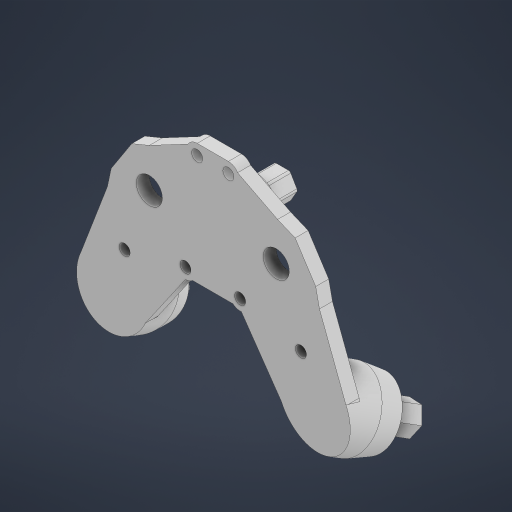
# Autodesk Inventor part: Neck_Baseplate_V2
Saved by Autodesk Inventor 2024 (Build 280153000, 153)
## iProperties
Created: 2025-09-27
Part Number: Neck_Baseplate_V2
Material: Generic
Document SubType Name: Modeling
Designer: kevin
Density: 1 g/cm^3
Appearance: Default
Author: kevin
Autodesk Inventor part; units mm, degrees
sketch "Sketch1" plane through (0, 0, 0) normal (0, 0, 1) x (1, 0, 0)
  line L0 (-6.0622, -7.1524) -> (-3.0311, -1.9024) projected
  line L1 (-3.0311, -1.9024) -> (3.0311, -1.9024) projected
  line L2 (3.0311, -1.9024) -> (6.0622, -7.1524) projected
  line L3 (6.0622, -7.1524) -> (3.0311, -12.4024) projected
  line L4 (3.0311, -12.4024) -> (-3.0311, -12.4024) projected
  line L5 (-3.0311, -12.4024) -> (-6.0622, -7.1524) projected
  circle A0 centre (0, -7.1524) radius 8.6602 projected
  line L6 (2.9156, -2.1024) -> (5.8312, -7.1524)
  line L7 (5.8312, -7.1524) -> (2.9156, -12.2024)
  line L8 (2.9156, -12.2024) -> (-2.9156, -12.2024)
  line L9 (-2.9156, -12.2024) -> (-5.8312, -7.1524)
  line L10 (-5.8312, -7.1524) -> (-2.9156, -2.1024)
  line L11 (-2.9156, -2.1024) -> (2.9156, -2.1024)
  point P0 (0, 0)
  dimension "d0" = 10.1
  constraints: 12 end point, 1 coincident, 1 parallel, 13 other
  measures "d0" distance between parallel lines of L8 L11
ref_plane "Work Plane1" through (-12.6537, -14.3928, -10.5) normal (0, 0, -1) x (0, 1, 0)
extrude "Extrusion1" add sketch "Sketch1" against normal up to surface (10.5 mm away) contours L6 L7 L8 L9 L10 L11
sketch "Sketch3" plane through (0, 0, 0) normal (0, 0, 1) x (1, 0, 0)
  circle A0 centre (0, -7.1524) radius 11.4859 projected
  arc A1 (11.152, -14.925) -> (11.152, 0.6202) centre (0, -7.1524) ccw projected
  circle A2 centre (0, -7.1524) radius 13.5934
  point P0 (0, 0)
  point P1 (11.152, 0.6202)
  point P2 (11.152, -14.925)
  constraints: 1 centre point, 1 coincident
extrude "Extrusion3" add sketch "Sketch3" along normal blind 11 contours A0 | A2 A1
ref_plane "Work Plane2" through (-43.2893, -53.3143, -8.1555) normal (0.2018432, 0.4641283, 0.862464) x (0.9791415, -0.1165411, -0.1664337)
sketch "Sketch5" plane through (-43.2893, -53.3143, -8.1555) normal (0.2018432, 0.4641283, 0.862464) x (0.9791415, -0.1165411, -0.1664337)
  line L0 (-6.0622, -7.1524) -> (-3.0311, -1.9024) projected
  line L1 (-3.0311, -1.9024) -> (3.0311, -1.9024) projected
  line L2 (3.0311, -1.9024) -> (6.0622, -7.1524) projected
  line L3 (6.0622, -7.1524) -> (3.0311, -12.4024) projected
  line L4 (3.0311, -12.4024) -> (-3.0311, -12.4024) projected
  line L5 (-3.0311, -12.4024) -> (-6.0622, -7.1524) projected
  circle A0 centre (0, -7.1524) radius 8.6602 projected
  line L6 (-2.9156, -12.2024) -> (-5.8312, -7.1524)
  line L7 (-5.8312, -7.1524) -> (-2.9156, -2.1024)
  line L8 (-2.9156, -2.1024) -> (2.9156, -2.1024)
  line L9 (2.9156, -2.1024) -> (5.8312, -7.1524)
  line L10 (5.8312, -7.1524) -> (2.9156, -12.2024)
  line L11 (2.9156, -12.2024) -> (-2.9156, -12.2024)
  point P0 (34.8157, 43.9226)
  dimension "d13" = 10.1
  constraints: 12 end point, 1 coincident, 1 parallel, 13 other
  measures "d13" distance between parallel lines of L8 L11
ref_plane "Work Plane3" through (-55.9189, -67.2082, -9.8974) normal (-0.2018432, -0.4641283, -0.862464) x (0.0232659, 0.8780678, -0.4779703)
extrude "Extrusion4" add sketch "Sketch5" against normal up to surface (10.5 mm away) contours L6 L7 L8 L9 L10 L11
fillet "Fillet1" radius 1 12 edges at (-47.2527, -57.2572, -11.1933) (-50.225, -61.3517, -8.2943) (-47.4877, -66.1257, -6.3658) (-41.5431, -57.9368, -12.1638) (-38.8058, -62.7108, -10.2354) (-41.7781, -66.8053, -7.3363) (-2.9156, -2.1024, -5.25) (-5.8312, -7.1524, -5.25) (-2.9156, -12.2024, -5.25) (2.9156, -2.1024, -5.25) (5.8312, -7.1524, -5.25) (2.9156, -12.2024, -5.25)
sketch "Sketch6" plane through (-43.2893, -53.3143, -8.1555) normal (0.2018432, 0.4641283, 0.862464) x (0.9791415, -0.1165411, -0.1664337)
  circle A0 centre (0, -7.1524) radius 11.4859 projected
  arc A1 (-11.152, 0.6202) -> (-11.152, -14.925) centre (0, -7.1524) ccw projected
  circle A2 centre (0, -7.1524) radius 13.5934
  point P0 (34.8157, 43.9226)
  point P1 (-11.152, -14.925)
  point P2 (-11.152, 0.6202)
  constraints: 1 centre point, 1 coincident
extrude "Extrusion5" add sketch "Sketch6" along normal blind 25.4 contours A0 | A2 A1
chamfer "Chamfer3" distance 2 angle 80 1 edges at (-32.7172, -67.7191, -2.8779) measured on face at (-43.6596, -66.527, -0.9586)
chamfer "Chamfer4" distance 2.75 angle 45 1 edges at (-34.2972, -66.5238, -3.1514)
chamfer "Chamfer5" distance 5 angle 45 1 edges at (-11.152, 0.6202, 0)
mirror "Mirror1" about plane through (0, 0, 0) normal (1, 0, 0) of "Extrusion4", "Extrusion5", "Chamfer4", "Chamfer3"
sketch "Sketch7" plane through (0, -7.1524, 11) normal (0, 0, 1) x (1, 0, 0)
  line L0 (62, -125.9339) -> (62, 49.4211) projected
  line L1 (-62, -125.9339) -> (62, -125.9339) projected
  line L2 (-62, 49.4211) -> (-62, -125.9339) projected
  line L3 (62, 49.4211) -> (-62, 49.4211) projected
  circle A0 centre (-35.0416, -115.806) radius 4 projected
  circle A1 centre (-0.3458, -115.806) radius 4 projected
  circle A2 centre (34.35, -115.806) radius 4 projected
  circle A3 centre (0, -77.5722) radius 2.1 projected
  circle A4 centre (-11, -67.3741) radius 2.1 projected
  circle A5 centre (11, -67.3741) radius 2.1 projected
  circle A6 centre (-6.25, 18.8827) radius 2.1 projected
  circle A7 centre (33.6286, -26.3451) radius 2.1 projected
  circle A8 centre (5.75, 18.8827) radius 2.1 projected
  circle A9 centre (-34.1286, -26.3451) radius 2.1 projected
  circle A10 centre (24.1373, -1.8845) radius 6.75 projected
  circle A11 centre (-24.6373, -1.8845) radius 6.75 projected
  circle A12 centre (-10.7484, -20.4549) radius 2.1 projected
  circle A13 centre (10.2484, -20.4549) radius 2.1 projected
  ellipse E0 centre (-38.3289, -40.6533) end of major axis (-25.8633, -46.0745) minor radius 11.7238 projected
  line L4 (0, -181.6265) -> (0, 141.5467)
  circle A14 centre (-6.25, 18.8827) radius 4.1
  circle A15 centre (5.75, 18.8827) radius 4.1
  line L5 (-6.25, 22.9827) -> (5.75, 22.9827)
  circle A16 centre (-24.6373, -1.8845) radius 8.75 construction
  line L6 (-9.7714, 20.9827) -> (-24.6373, 13.1086)
  line L7 (-24.6373, 13.1086) -> (-31.3873, 10.3122)
  line L8 (-31.3873, 10.3122) -> (-39.29, -1.8845)
  line L9 (-39.29, -1.8845) -> (-40.7219, -8.6345)
  line L10 (-40.7219, -8.6345) -> (-50.9767, -35.6799)
  arc A17 (-10.7484, -24.5549) -> (-8.0196, -23.5149) centre (-10.7484, -20.4549) ccw
  arc A18 (7.5196, -23.5149) -> (10.7288, -24.5267) centre (10.2484, -20.4549) ccw
  line L11 (24.6373, 13.1086) -> (31.3873, 10.3122)
  line L12 (31.3873, 10.3122) -> (39.29, -1.8845)
  line L13 (39.29, -1.8845) -> (40.7219, -8.6345)
  line L14 (40.7219, -8.6345) -> (50.9767, -35.6799)
  ellipse E1 centre (38.3289, -40.6533) end of major axis (25.8633, -46.0745) minor radius 11.7238 projected
  line L15 (-26.3694, -47.081) -> (-10.7484, -24.5549)
  line L16 (-8.0196, -23.5149) -> (7.5196, -23.5149)
  line L17 (26.3694, -47.081) -> (10.7288, -24.5267)
  line L18 (-9.7714, 20.9827) -> (18.0265, 20.9827) construction
  line L19 (9.2714, 20.9827) -> (24.6373, 13.1086)
  circle A19 centre (-24.6373, -1.8845) radius 5
  circle A20 centre (24.1373, -1.8845) radius 5
  point P0 (0, 7.1524)
  point P1 (10.7484, -24.5549)
  point P2 (26.3694, -47.081)
  dimension "d28" = 2
  dimension "d29" = 2
  dimension "d30" = 2
  dimension "d31" = 2
  dimension "d32" = 2
  dimension "d37" = 10
  dimension "d38" = 10
  constraints: 32 end point, 8 point on circle, 7 centre point, 7 symmetric about line, 2 coincident, 2 horizontal, 2 point on line, 1 tangent, 1 vertical, 7 other
  measures "d28" radial gap between concentric circles of A6 A14
  measures "d29" radial gap between concentric circles of A8 A15
  measures "d30" radial gap between concentric circles of A11 A16
  measures "d31" radial gap between concentric circles of A12 A17
  measures "d32" radial gap between concentric circles of A13 A18
  measures "d37" diameter of A19
  measures "d38" diameter of A20
extrude "Extrusion6" add sketch "Sketch7" along normal blind 5 contours L5 A15 L19 L11 L12 L13 L14 E1 L17 A18 L16 L4 | L4 L16 A17 L15 E0 L10 L9 L8 L7 L6 A14 L5 | A14 | A15 | E0 | E1 | A10 | A11
sketch "Sketch8" plane through (0, -7.1524, 16) normal (0, 0, 1) x (1, 0, 0)
  line L0 (-69.201, -87.0843) -> (64.7933, -87.0843)
  line L1 (64.7933, -87.0843) -> (64.7933, 51.6702)
  line L2 (64.7933, 51.6702) -> (-69.201, 51.6702)
  line L3 (-69.201, 51.6702) -> (-69.201, -87.0843)
  point P0 (0, 7.1524)
  constraints: 8 end point, 2 parallel, 1 horizontal, 1 perpendicular
extrude "Extrusion7" cut sketch "Sketch8" along normal blind 11
body "Solid1"
